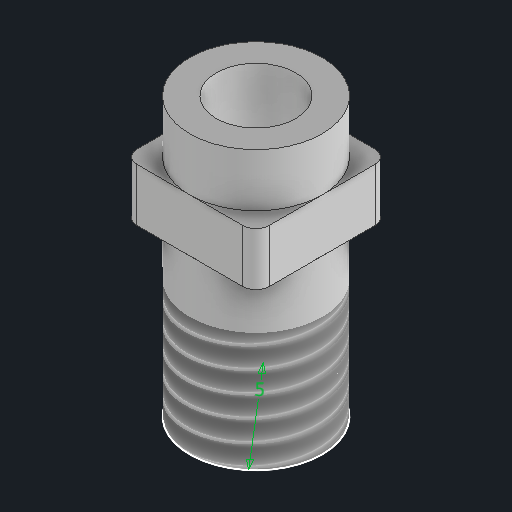
# Autodesk Inventor part: RadAdapterSchaft
Saved by Autodesk Inventor 2026.1 (Build 301233000, 233)
## iProperties
Created: 2025-10-13
Part Number: RadAdapterSchaft
Material: Generisch
Document SubType Name: Modeling
Designer: JurijLenz
Density: 1 g/cm^3
Appearance: Vorgabe
Author: JurijLenz
Autodesk Inventor part; units mm, degrees
ref_plane "YZ Plane" through (0, 0, 0) normal (1, 0, 0) x (0, 1, 0)
ref_plane "XZ Plane" through (0, 0, 0) normal (0, 1, 0) x (-1, 0, 0)
sketch "Skizze1" plane through (0, 0, 0) normal (0, 0, 1) x (1, 0, 0)
  circle A0 centre (0, 0) radius 2.5
  dimension "d1" = 5
  constraints: 2 coincident, 1 centre point
  measures "d1" diameter of A0
extrude "Extrusion1" add sketch "Skizze1" along normal blind 10.5
thread "Gewinde1" size "M5x0.8" class "6g" standard "ANSI Metric M Profile" length 4.5
sketch "Skizze2" plane through (0, 0, 10.5) normal (0, 0, 1) x (1, 0, 0)
  circle A0 centre (0, 0) radius 1.5 projected
ref_plane "Arbeitsebene1" through (0, 0, 8.5) normal (0, 0, -1) x (-1, 0, 0)
sketch "Skizze3" plane through (0, 0, 8.5) normal (0, 0, -1) x (-1, 0, 0)
  line L0 (-2.5, -2.5) -> (2.5, -2.5)
  line L1 (2.5, -2.5) -> (2.5, 2.5)
  line L2 (2.5, 2.5) -> (-2.5, 2.5)
  line L3 (-2.5, 2.5) -> (-2.5, -2.5)
  line L4 (-2.5, -2.5) -> (2.5, 2.5) construction
  line L5 (2.5, -2.5) -> (-2.5, 2.5) construction
  point P0 (0, 0)
  constraints: 12 end point, 2 midpoint, 2 parallel, 1 horizontal, 1 perpendicular
extrude "Extrusion3" add sketch "Skizze3" along normal blind 2
fillet "Rundung2" radius 0.5 4 edges at (2.5, -2.5, 7.5) (2.5, 2.5, 7.5) (-2.5, -2.5, 7.5) (-2.5, 2.5, 7.5)
hole "Bohrung2" at (0, 0, 10.5) direction (0, 0, -1) diameter 3 end through all
